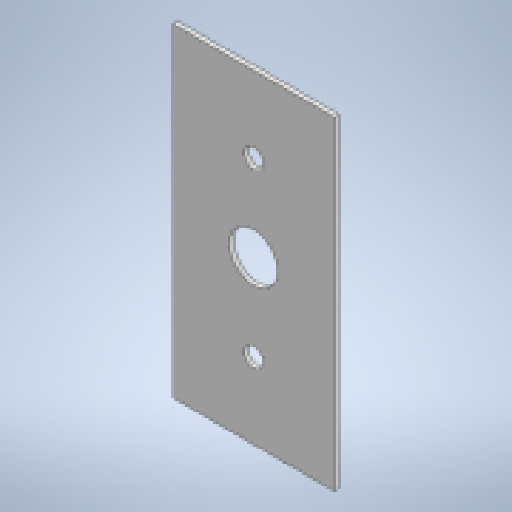
# Autodesk Inventor part: kosisita
Saved by Autodesk Inventor 2024 (Build 280153000, 153)
## iProperties
Created: 2024-07-10
Part Number: kosisita
Material: 一般
Document SubType Name: Modeling
Designer: right
Density: 1 g/cm^3
Appearance: 既定
Author: right
Autodesk Inventor part; units mm, degrees
ref_plane "YZ Plane" through (0, 0, 0) normal (1, 0, 0) x (0, 1, 0)
ref_plane "XZ Plane" through (0, 0, 0) normal (0, 1, 0) x (-1, 0, 0)
ref_plane "XY Plane" through (0, 0, 0) normal (0, 0, 1) x (1, 0, 0)
sketch "スケッチ1" plane through (0, 0, 0) normal (0, 0, 1) x (1, 0, 0)
  circle A0 centre (0, 0) radius 1.75 projected
  circle A1 centre (0, 0) radius 3
  circle A2 centre (0, -53.1322) radius 1.75 projected
  circle A3 centre (0, -53.1322) radius 3
  line L0 (0, 0) -> (0, -53.1322) construction
  circle A4 centre (0, -26.5661) radius 7.5
  line L1 (25, 29.4339) -> (-25, 29.4339)
  line L2 (-25, 29.4339) -> (-25, -82.5661)
  line L3 (-25, -82.5661) -> (25, -82.5661)
  line L4 (25, -82.5661) -> (25, 29.4339)
  line L5 (25, 29.4339) -> (-25, -82.5661) construction
  line L6 (-25, 29.4339) -> (25, -82.5661) construction
  line L7 (25, -26.5661) -> (0, -26.5661) construction
  circle A5 centre (-10, -79.6778) radius 0.7835 projected
  point P0 (0, 0)
  point P1 (5, 29.4339)
  point P2 (-5, 29.4339)
  dimension "d0" = 6
  dimension "d1" = 6
  dimension "d2" = 15
  dimension "d4" = 50
  dimension "d14" = 112
  constraints: 16 end point, 4 midpoint, 3 centre point, 2 coincident, 2 horizontal, 2 parallel, 2 point on line, 1 perpendicular, 1 vertical
  measures "d0" diameter of A1
  measures "d1" diameter of A3
  measures "d2" diameter of A4
  measures "d4" distance between parallel lines of L2 L4
  measures "d14" distance of L1.end L2.end
extrude "押し出し1" add sketch "スケッチ1" along normal blind 1.5 contours L4 L3 L2 L1 | A5
sketch "スケッチ2" plane through (0, 0, 1.5) normal (0, 0, 1) x (1, 0, 0)
  line L0 (-5, -78.1778) -> (5, -78.1778) projected
  line L1 (-5, -81.1778) -> (5, -81.1778) projected
  line L2 (-5, -81.1778) -> (-5, -78.1778) projected
  line L3 (5, -81.1778) -> (5, -78.1778) projected
  circle A0 centre (-10, -79.6778) radius 0.7835 projected
  circle A1 centre (10, -79.6778) radius 0.7835 projected
  line L4 (5, 25.0456) -> (-5, 25.0456) projected
  line L5 (5, 28.0456) -> (-5, 28.0456) projected
  line L6 (-5, 28.0456) -> (-5, 25.0456) projected
  line L7 (5, 28.0456) -> (5, 25.0456) projected
  circle A2 centre (-10, 26.5456) radius 0.7835 projected
  circle A3 centre (10, 26.5456) radius 0.7835 projected
  circle A4 centre (3.9, -78.1778) radius 1.1
  line L8 (0, -78.1778) -> (0, -81.1778) construction
  line L9 (0, -79.6778) -> (-5, -79.6778) construction
  circle A5 centre (3.9, -81.1778) radius 1.1
  circle A6 centre (-3.9, -78.1778) radius 1.1
  circle A7 centre (-3.9, -81.1778) radius 1.1
  line L10 (-25, 29.4339) -> (-25, -82.5661) construction
  line L11 (-25, -26.5661) -> (25, -26.5661) construction
  line L12 (25, -82.5661) -> (25, 29.4339) construction
  circle A8 centre (3.9, 25.0456) radius 1.1
  circle A9 centre (3.9, 28.0456) radius 1.1
  circle A10 centre (-3.9, 28.0456) radius 1.1
  circle A11 centre (-3.9, 25.0456) radius 1.1
  circle A12 centre (-10, -79.6778) radius 1.1
  circle A13 centre (10, -79.6778) radius 1.1
  circle A14 centre (-10, 26.5456) radius 1.1
  circle A15 centre (10, 26.5456) radius 1.1
  point P0 (0, 0)
  point P1 (2.8, 25.0456)
  point P2 (-2.8, 25.0456)
  point P3 (-2.8, 28.0456)
  point P4 (2.8, -81.1778)
  point P5 (2.8, -78.1778)
  point P6 (-2.8, -81.1778)
  point P7 (-2.8, -78.1778)
  point P8 (2.8, 28.0456)
  dimension "d17" = 2.2
  dimension "d18" = 2.2
  dimension "d19" = 2.2
  dimension "d20" = 2.2
  dimension "d21" = 2.2
  constraints: 11 centre point, 7 symmetric about line, 6 end point, 6 midpoint, 4 coincident, 1 point on line, 10 other
  measures "d18" diameter of A12
  measures "d19" diameter of A13
  measures "d20" diameter of A14
  measures "d21" diameter of A15
extrude "押し出し2" cut sketch "スケッチ2" against normal through all contours A6 L0 | A6 L0 A4 L3 A5 L1 A7 L2 | L0 A6 | A7 L1 | L1 A7 | A4 L0 | L0 A4 | A5 L1 | L1 A5 | A0 | A1 | A11 L4 | A11 L6 A10 L5 A9 L7 A8 L4 | L4 A11 | A8 L4 | L4 A8 | A10 L5 | L5 A10 | A9 L5 | L5 A9 | A2 | A3 | A12 | A13 | A14 | A15
